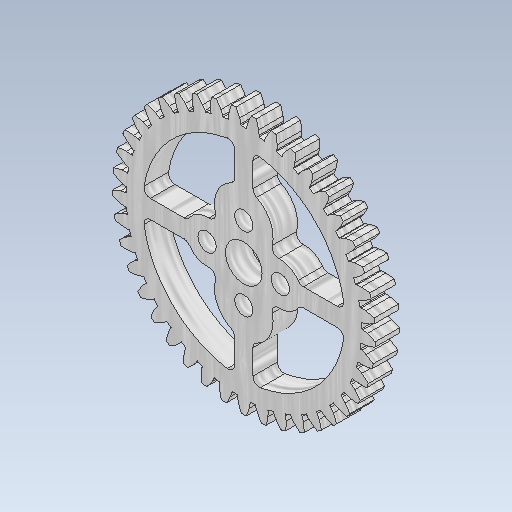
# Autodesk Inventor part: m1歯数41ギアd6t4
Saved by Autodesk Inventor 2020.2 (Build 242310000, 310)
## iProperties
Created: 2020-03-15
Part Number: m1歯数41ギアd6t4
Material: アルミニウム 7075
Document SubType Name: Modeling
Designer: aoyam
Density: 2.81 g/cm^3
Appearance: サテン - ブラシ仕上げ 重厚
Mass: 7.9651 g
Surface Area: 34.7064 cm^2
Volume: 2.83456 cm^3
Author: aoyam
Autodesk Inventor part; units mm, degrees
ref_plane "YZ Plane" through (0, 0, 0) normal (1, 0, 0) x (0, 1, 0)
ref_plane "XZ Plane" through (0, 0, 0) normal (0, 1, 0) x (-1, 0, 0)
ref_plane "XY Plane" through (0, 0, 0) normal (0, 0, 1) x (1, 0, 0)
sketch "スケッチ1" plane through (0, 0, 0) normal (0, 0, 1) x (1, 0, 0)
  arc A0 (3.2074, 20.8841) -> (3.1784, 20.6559) centre (4.8478, 20.5595) ccw
  arc A1 (3.4025, 21.5932) -> (3.2074, 20.8841) centre (7.7041, 20.0288) ccw
  arc A2 (3.993, 22.8602) -> (3.4025, 21.5932) centre (10.7748, 18.928) ccw
  arc A3 (2.2767, 20.6559) -> (2.2477, 20.8841) centre (0.6073, 20.5595) ccw
  arc A4 (2.2477, 20.8841) -> (2.0526, 21.5932) centre (-2.249, 20.0288) ccw
  arc A5 (2.0526, 21.5932) -> (1.4621, 22.8602) centre (-5.3197, 18.928) ccw
  arc A6 (3.1781, 20.6422) -> (2.277, 20.6422) centre (2.7276, 1.3974) ccw
  arc A7 (1.4621, 22.8602) -> (0.7019, 22.8018) centre (2.7276, 1.3974) ccw
  line L0 (3.1781, 20.6422) -> (3.1784, 20.6559)
  line L1 (2.277, 20.6422) -> (2.2767, 20.6559)
  arc A8 (0.2272, 20.729) -> (0.2334, 20.499) centre (1.8978, 20.6586) ccw
  arc A9 (0.2351, 20.4854) -> (-0.6554, 20.3478) centre (2.7276, 1.3974) ccw
  line L2 (0.2351, 20.4854) -> (0.2334, 20.499)
  line L3 (-0.6554, 20.3478) -> (-0.6578, 20.3613)
  arc A10 (-0.6578, 20.3613) -> (-0.7213, 20.5824) centre (-2.2929, 20.0113) ccw
  arc A11 (0.3117, 21.4596) -> (0.2272, 20.729) centre (4.8017, 20.5701) ccw
  arc A12 (-0.7213, 20.5824) -> (-1.0223, 21.2535) centre (-5.0348, 19.0507) ccw
  arc A13 (0.7019, 22.8018) -> (0.3117, 21.4596) centre (8.0044, 19.9509) ccw
  arc A14 (-1.0223, 21.2535) -> (-1.7994, 22.4155) centre (-7.9014, 17.4941) ccw
  arc A15 (-1.7994, 22.4155) -> (-2.5417, 22.2417) centre (2.7276, 1.3974) ccw
  arc A16 (-2.6944, 20.1207) -> (-2.6532, 19.8944) centre (-1.0326, 20.3062) ccw
  arc A17 (-2.6494, 19.8812) -> (-3.5085, 19.6093) centre (2.7276, 1.3974) ccw
  line L4 (-2.6494, 19.8812) -> (-2.6532, 19.8944)
  line L5 (-3.5085, 19.6093) -> (-3.513, 19.6223)
  arc A18 (-3.513, 19.6223) -> (-3.6095, 19.8311) centre (-5.0755, 19.0268) ccw
  arc A19 (-2.7225, 20.8557) -> (-2.6944, 20.1207) centre (1.8507, 20.662) ccw
  arc A20 (-3.6095, 19.8311) -> (-4.0094, 20.4484) centre (-7.6385, 17.6589) ccw
  arc A21 (-2.5417, 22.2417) -> (-2.7225, 20.8557) centre (5.1104, 20.539) ccw
  arc A22 (-4.0094, 20.4484) -> (-4.9547, 21.4781) centre (-10.234, 15.683) ccw
  arc A23 (-4.9547, 21.4781) -> (-5.6618, 21.1931) centre (2.7276, 1.3974) ccw
  arc A24 (-5.489, 19.0736) -> (-5.4137, 18.8562) centre (-3.875, 19.5106) ccw
  arc A25 (-5.4079, 18.8438) -> (-6.2155, 18.444) centre (2.7276, 1.3974) ccw
  line L6 (-5.4079, 18.8438) -> (-5.4137, 18.8562)
  line L7 (-6.2155, 18.444) -> (-6.2219, 18.4561)
  arc A26 (-6.2219, 18.4561) -> (-6.3491, 18.6477) centre (-7.6751, 17.6291) ccw
  arc A27 (-5.6289, 19.7957) -> (-5.489, 19.0736) centre (-1.0797, 20.3024) ccw
  arc A28 (-6.3491, 18.6477) -> (-6.8386, 19.1967) centre (-9.9994, 15.886) ccw
  arc A29 (-5.6618, 21.1931) -> (-5.6289, 19.7957) centre (2.1605, 20.6784) ccw
  arc A30 (-6.8386, 19.1967) -> (-7.93, 20.0701) centre (-12.2627, 13.537) ccw
  arc A31 (-7.93, 20.0701) -> (-8.5853, 19.6805) centre (2.7276, 1.3974) ccw
  arc A32 (-8.091, 17.6122) -> (-7.9834, 17.4089) centre (-6.5626, 18.2905) ccw
  arc A33 (-7.9758, 17.3975) -> (-8.7128, 16.879) centre (2.7276, 1.3974) ccw
  line L8 (-7.9758, 17.3975) -> (-7.9834, 17.4089)
  line L9 (-8.7128, 16.879) -> (-8.721, 16.8901)
  arc A34 (-8.721, 16.8901) -> (-8.876, 17.06) centre (-10.031, 15.8509) ccw
  arc A35 (-8.3394, 18.3045) -> (-8.091, 17.6122) centre (-3.9209, 19.4997) ccw
  arc A36 (-8.876, 17.06) -> (-9.4435, 17.5279) centre (-12.0619, 13.7734) ccw
  arc A37 (-8.5853, 19.6805) -> (-8.3394, 18.3045) centre (-0.7761, 20.3659) ccw
  arc A38 (-9.4435, 17.5279) -> (-10.6554, 18.2244) centre (-13.9401, 11.1065) ccw
  arc A39 (-10.6554, 18.2244) -> (-11.2436, 17.7393) centre (2.7276, 1.3974) ccw
  arc A40 (-10.4393, 15.7708) -> (-10.302, 15.5862) centre (-9.0324, 16.6744) ccw
  arc A41 (-10.2927, 15.5761) -> (-10.942, 14.9512) centre (2.7276, 1.3974) ccw
  line L10 (-10.2927, 15.5761) -> (-10.302, 15.5862)
  line L11 (-10.942, 14.9512) -> (-10.9517, 14.9609)
  arc A42 (-10.9517, 14.9609) -> (-11.1309, 15.1052) centre (-12.0877, 13.7339) ccw
  arc A43 (-10.7906, 16.417) -> (-10.4393, 15.7708) centre (-6.6063, 18.2726) ccw
  arc A44 (-11.1309, 15.1052) -> (-11.7632, 15.4809) centre (-13.7777, 11.3708) ccw
  arc A45 (-11.2436, 17.7393) -> (-10.7906, 16.417) centre (-3.6305, 19.6088) ccw
  arc A46 (-11.7632, 15.4809) -> (-13.0672, 15.9843) centre (-15.2269, 8.4484) ccw
  arc A47 (-13.0672, 15.9843) -> (-13.5744, 15.4151) centre (2.7276, 1.3974) ccw
  arc A48 (-12.4791, 13.5924) -> (-12.3152, 13.431) centre (-11.2266, 14.7002) ccw
  arc A49 (-12.3045, 13.4224) -> (-12.8508, 12.7058) centre (2.7276, 1.3974) ccw
  line L12 (-12.3045, 13.4224) -> (-12.3152, 13.431)
  line L13 (-12.8508, 12.7058) -> (-12.8619, 12.7138)
  arc A50 (-12.8619, 12.7138) -> (-13.061, 12.8291) centre (-13.7973, 11.3278) ccw
  arc A51 (-12.9249, 14.1774) -> (-12.4791, 13.5924) centre (-9.0729, 16.65) ccw
  arc A52 (-13.061, 12.8291) -> (-13.7432, 13.1039) centre (-15.1067, 8.7344) ccw
  arc A53 (-13.5744, 15.4151) -> (-12.9249, 14.1774) centre (-6.336, 18.4248) ccw
  arc A54 (-13.7432, 13.1039) -> (-15.1088, 13.4023) centre (-16.0928, 5.625) ccw
  arc A55 (-15.1088, 13.4023) -> (-15.5232, 12.7623) centre (2.7276, 1.3974) ccw
  arc A56 (-14.1624, 11.1282) -> (-13.9758, 10.9937) centre (-13.0937, 12.4142) ccw
  arc A57 (-13.9639, 10.9868) -> (-14.3944, 10.1952) centre (2.7276, 1.3974) ccw
  line L14 (-13.9639, 10.9868) -> (-13.9758, 10.9937)
  line L15 (-14.3944, 10.1952) -> (-14.4066, 10.2015)
  arc A58 (-14.4066, 10.2015) -> (-14.621, 10.285) centre (-15.1195, 8.6889) ccw
  arc A59 (-14.6923, 11.6383) -> (-14.1624, 11.1282) centre (-11.2629, 14.67) ccw
  arc A60 (-14.621, 10.285) -> (-15.3371, 10.4524) centre (-16.0177, 5.926) ccw
  arc A61 (-15.5232, 12.7623) -> (-14.6923, 11.6383) centre (-8.8289, 16.8417) ccw
  arc A62 (-15.3371, 10.4524) -> (-16.7323, 10.5389) centre (-16.5176, 2.7026) ccw
  arc A63 (-16.7323, 10.5389) -> (-17.0441, 9.8432) centre (2.7276, 1.3974) ccw
  arc A64 (-15.4499, 8.4359) -> (-15.2449, 8.3314) centre (-14.59, 9.87) ccw
  arc A65 (-15.2321, 8.3265) -> (-15.5367, 7.4784) centre (2.7276, 1.3974) ccw
  line L16 (-15.2321, 8.3265) -> (-15.2449, 8.3314)
  line L17 (-15.5367, 7.4784) -> (-15.5497, 7.4828)
  arc A66 (-15.5497, 7.4828) -> (-15.7743, 7.5326) centre (-16.0233, 5.8791) ccw
  arc A67 (-16.0514, 8.8592) -> (-15.4499, 8.4359) centre (-13.125, 12.3788) ccw
  arc A68 (-15.7743, 7.5326) -> (-16.5077, 7.5887) centre (-16.4893, 3.0115) ccw
  arc A69 (-17.0441, 9.8432) -> (-16.0514, 8.8592) centre (-11.0511, 14.8966) ccw
  arc A70 (-16.5077, 7.5887) -> (-17.8996, 7.4612) centre (-16.4912, -0.2505) ccw
  arc A71 (-17.8996, 7.4612) -> (-18.1017, 6.7261) centre (2.7276, 1.3974) ccw
  arc A72 (-16.3113, 5.5786) -> (-16.0928, 5.5067) centre (-15.6804, 7.1272) ccw
  arc A73 (-16.0794, 5.5038) -> (-16.2509, 4.6191) centre (2.7276, 1.3974) ccw
  line L18 (-16.0794, 5.5038) -> (-16.0928, 5.5067)
  line L19 (-16.2509, 4.6191) -> (-16.2644, 4.6214)
  arc A74 (-16.2644, 4.6214) -> (-16.494, 4.6364) centre (-16.4877, 2.9643) ccw
  arc A75 (-16.9703, 5.9051) -> (-16.3113, 5.5786) centre (-14.6155, 9.8302) ccw
  arc A76 (-16.494, 4.6364) -> (-17.2273, 4.5799) centre (-16.5105, 0.0591) ccw
  arc A77 (-18.1017, 6.7261) -> (-16.9703, 5.9051) centre (-12.9502, 12.6351) ccw
  arc A78 (-17.2273, 4.5799) -> (-18.5835, 4.2414) centre (-16.0145, -3.1649) ccw
  arc A79 (-18.5835, 4.2414) -> (-18.671, 3.4841) centre (2.7276, 1.3974) ccw
  arc A80 (-16.7264, 2.6234) -> (-16.4995, 2.5856) centre (-16.3393, 4.2501) ccw
  arc A81 (-16.4858, 2.5848) -> (-16.5203, 1.6843) centre (2.7276, 1.3974) ccw
  line L20 (-16.4858, 2.5848) -> (-16.4995, 2.5856)
  line L21 (-16.5203, 1.6843) -> (-16.534, 1.6845)
  arc A82 (-16.534, 1.6845) -> (-16.7632, 1.6643) centre (-16.5017, 0.0127) ccw
  arc A83 (-17.4276, 2.8454) -> (-16.7264, 2.6234) centre (-15.6995, 7.084) ccw
  arc A84 (-16.7632, 1.6643) -> (-17.4793, 1.4965) centre (-16.0807, -2.8619) ccw
  arc A85 (-18.671, 3.4841) -> (-17.4276, 2.8454) centre (-14.4819, 10.1102) ccw
  arc A86 (-17.4793, 1.4965) -> (-18.7679, 0.955) centre (-15.0984, -5.9724) ccw
  arc A87 (-18.7679, 0.955) -> (-18.7387, 0.1931) centre (2.7276, 1.3974) ccw
  arc A88 (-16.6856, -0.3606) -> (-16.4555, -0.3633) centre (-16.5513, 1.3061) ccw
  arc A89 (-16.4419, -0.362) -> (-16.3385, -1.2572) centre (2.7276, 1.3974) ccw
  line L22 (-16.4419, -0.362) -> (-16.4555, -0.3633)
  line L23 (-16.3385, -1.2572) -> (-16.3521, -1.2591)
  arc A90 (-16.3521, -1.2591) -> (-16.5755, -1.3141) centre (-16.065, -2.9064) ccw
  arc A91 (-17.4124, -0.2482) -> (-16.6856, -0.3606) centre (-16.3516, 4.2045) ccw
  arc A92 (-16.5755, -1.3141) -> (-17.2576, -1.5892) centre (-15.2101, -5.683) ccw
  arc A93 (-18.7387, 0.1931) -> (-17.4124, -0.2482) centre (-15.6102, 7.3811) ccw
  arc A94 (-17.2576, -1.5892) -> (-18.4484, -2.3211) centre (-13.7645, -8.6071) ccw
  arc A95 (-18.4484, -2.3211) -> (-18.3033, -3.0696) centre (2.7276, 1.3974) ccw
  arc A96 (-16.1897, -3.3034) -> (-15.9619, -3.2709) centre (-16.3114, -1.6357) ccw
  arc A97 (-15.9486, -3.2676) -> (-15.7099, -4.1365) centre (2.7276, 1.3974) ccw
  line L24 (-15.9486, -3.2676) -> (-15.9619, -3.2709)
  line L25 (-15.7099, -4.1365) -> (-15.723, -4.1405)
  arc A98 (-15.723, -4.1405) -> (-15.9353, -4.2289) centre (-15.1878, -5.7246) ccw
  arc A99 (-16.9252, -3.3033) -> (-16.1897, -3.3034) centre (-16.5565, 1.2592) ccw
  arc A100 (-15.9353, -4.2289) -> (-16.5675, -4.6049) centre (-13.9191, -8.3382) ccw
  arc A101 (-18.3033, -3.0696) -> (-16.9252, -3.3033) centre (-16.3087, 4.5117) ccw
  arc A102 (-16.5675, -4.6049) -> (-17.6326, -5.51) centre (-12.044, -11.0074) ccw
  arc A103 (-17.6326, -5.51) -> (-17.3749, -6.2275) centre (2.7276, 1.3974) ccw
  arc A104 (-15.2504, -6.136) -> (-15.0303, -6.0692) centre (-15.6253, -4.5065) ccw
  arc A105 (-15.0176, -6.0638) -> (-14.649, -6.8861) centre (2.7276, 1.3974) ccw
  line L26 (-15.0176, -6.0638) -> (-15.0303, -6.0692)
  line L27 (-14.649, -6.8861) -> (-14.6614, -6.892)
  arc A106 (-14.6614, -6.892) -> (-14.8578, -7.0118) centre (-13.8906, -8.3759) ccw
  arc A107 (-15.9773, -6.2482) -> (-15.2504, -6.136) centre (-16.3094, -1.6829) ccw
  arc A108 (-14.8578, -7.0118) -> (-15.4251, -7.4799) centre (-12.2378, -10.7652) ccw
  arc A109 (-17.3749, -6.2275) -> (-15.9773, -6.2482) centre (-16.561, 1.5693) ccw
  arc A110 (-15.4251, -7.4799) -> (-16.3396, -8.537) centre (-9.9773, -13.1169) ccw
  arc A111 (-16.3396, -8.537) -> (-15.9754, -9.2068) centre (2.7276, 1.3974) ccw
  arc A112 (-13.8897, -8.7921) -> (-13.6824, -8.6924) centre (-14.5089, -7.2388) ccw
  arc A113 (-13.6707, -8.6852) -> (-13.1809, -9.4416) centre (2.7276, 1.3974) ccw
  line L28 (-13.6707, -8.6852) -> (-13.6824, -8.6924)
  line L29 (-13.1809, -9.4416) -> (-13.1922, -9.4493)
  arc A114 (-13.1922, -9.4493) -> (-13.368, -9.5977) centre (-12.204, -10.7981) ccw
  arc A115 (-14.591, -9.0138) -> (-13.8897, -8.7921) centre (-15.616, -4.5528) ccw
  arc A116 (-13.368, -9.5977) -> (-13.8572, -10.1469) centre (-10.2058, -12.9071) ccw
  arc A117 (-15.9754, -9.2068) -> (-14.591, -9.0138) centre (-16.3612, -1.3771) ccw
  arc A118 (-13.8572, -10.1469) -> (-14.5996, -11.3312) centre (-7.6128, -14.8861) ccw
  arc A119 (-14.5996, -11.3312) -> (-14.1375, -11.9375) centre (2.7276, 1.3974) ccw
  arc A120 (-12.1395, -11.2093) -> (-11.9499, -11.0791) centre (-12.9886, -9.7688) ccw
  arc A121 (-11.9394, -11.0702) -> (-11.3399, -11.7429) centre (2.7276, 1.3974) ccw
  line L30 (-11.9394, -11.0702) -> (-11.9499, -11.0791)
  line L31 (-11.3399, -11.7429) -> (-11.3499, -11.7523)
  arc A122 (-11.3499, -11.7523) -> (-11.501, -11.9258) centre (-10.1674, -12.9345) ccw
  arc A123 (-12.7987, -11.5355) -> (-12.1395, -11.2093) centre (-14.4928, -7.2832) ccw
  arc A124 (-11.501, -11.9258) -> (-11.9006, -12.5432) centre (-7.8707, -14.7137) ccw
  arc A125 (-14.1375, -11.9375) -> (-12.7987, -11.5355) centre (-15.7139, -4.2584) ccw
  arc A126 (-11.9006, -12.5432) -> (-12.4536, -13.827) centre (-5.0059, -16.2738) ccw
  arc A127 (-12.4536, -13.827) -> (-11.9042, -14.3557) centre (2.7276, 1.3974) ccw
  arc A128 (-10.0409, -13.331) -> (-9.8733, -13.1734) centre (-11.0999, -12.037) ccw
  arc A129 (-9.8644, -13.163) -> (-9.1692, -13.7363) centre (2.7276, 1.3974) ccw
  line L32 (-9.8644, -13.163) -> (-9.8733, -13.1734)
  line L33 (-9.1692, -13.7363) -> (-9.1776, -13.7471)
  arc A130 (-9.1776, -13.7471) -> (-9.3004, -13.9416) centre (-7.8285, -14.7349) ccw
  arc A131 (-10.6426, -13.754) -> (-10.0409, -13.331) centre (-12.9659, -9.8101) ccw
  arc A132 (-9.3004, -13.9416) -> (-9.6012, -14.6128) centre (-5.2871, -16.1427) ccw
  arc A133 (-11.9042, -14.3557) -> (-10.6426, -13.754) centre (-14.6345, -7.0072) ccw
  arc A134 (-9.6012, -14.6128) -> (-9.9516, -15.966) centre (-2.2178, -17.2472) ccw
  arc A135 (-9.9516, -15.966) -> (-9.3281, -16.4046) centre (2.7276, 1.3974) ccw
  arc A136 (-7.643, -15.1074) -> (-7.5014, -14.9261) centre (-8.8871, -13.9903) ccw
  arc A137 (-7.4942, -14.9145) -> (-6.7196, -15.375) centre (2.7276, 1.3974) ccw
  line L34 (-7.4942, -14.9145) -> (-7.5014, -14.9261)
  line L35 (-6.7196, -15.375) -> (-6.7263, -15.3869)
  arc A138 (-6.7263, -15.3869) -> (-6.818, -15.5979) centre (-5.2422, -16.1572) ccw
  arc A139 (-8.173, -15.6173) -> (-7.643, -15.1074) centre (-11.0711, -12.0744) ccw
  arc A140 (-6.818, -15.5979) -> (-7.0127, -16.3072) centre (-2.5157, -17.1606) ccw
  arc A141 (-9.3281, -16.4046) -> (-8.173, -15.6173) centre (-13.148, -9.559) ccw
  arc A142 (-7.0127, -16.3072) -> (-7.1525, -17.698) centre (0.6862, -17.7836) ccw
  arc A143 (-7.1525, -17.698) -> (-6.4693, -18.0362) centre (2.7276, 1.3974) ccw
  arc A144 (-5.002, -16.4971) -> (-4.8898, -16.2963) centre (-6.4021, -15.5829) ccw
  arc A145 (-4.8844, -16.2837) -> (-4.0486, -16.6205) centre (2.7276, 1.3974) ccw
  line L36 (-4.8844, -16.2837) -> (-4.8898, -16.2963)
  line L37 (-4.0486, -16.6205) -> (-4.0534, -16.6333)
  arc A146 (-4.0534, -16.6333) -> (-4.1118, -16.8559) centre (-2.4691, -17.168) ccw
  arc A147 (-5.448, -17.0819) -> (-5.002, -16.4971) centre (-8.8529, -14.0228) ccw
  arc A148 (-4.1118, -16.8559) -> (-4.196, -17.5865) centre (0.3786, -17.7435) ccw
  arc A149 (-6.4693, -18.0362) -> (-5.448, -17.0819) centre (-11.2895, -11.854) ccw
  arc A150 (-4.196, -17.5865) -> (-4.1219, -18.9824) centre (3.6381, -17.8704) ccw
  arc A151 (-4.1219, -18.9824) -> (-3.395, -19.2124) centre (2.7276, 1.3974) ccw
  arc A152 (-2.1798, -17.4673) -> (-2.0996, -17.2517) centre (-3.703, -16.7775) ccw
  arc A153 (-2.0961, -17.2384) -> (-1.2187, -17.4437) centre (2.7276, 1.3974) ccw
  line L38 (-2.0961, -17.2384) -> (-2.0996, -17.2517)
  line L39 (-1.2187, -17.4437) -> (-1.2215, -17.4571)
  arc A154 (-1.2215, -17.4571) -> (-1.2453, -17.686) centre (0.4258, -17.7437) ccw
  arc A155 (-2.5313, -18.1133) -> (-2.1798, -17.4673) centre (-6.3633, -15.6099) ccw
  arc A156 (-1.2453, -17.686) -> (-1.217, -18.4209) centre (3.328, -17.8777) ccw
  arc A157 (-3.395, -19.2124) -> (-2.5313, -18.1133) centre (-9.1024, -13.8384) ccw
  arc A158 (-1.217, -18.4209) -> (-0.9306, -19.7891) centre (6.5687, -17.5056) ccw
  arc A159 (-0.9306, -19.7891) -> (-0.1772, -19.9054) centre (2.7276, 1.3974) ccw
  arc A160 (0.7574, -17.9953) -> (0.8038, -17.77) centre (-0.8533, -17.5461) ccw
  arc A161 (0.8051, -17.7563) -> (1.7036, -17.8253) centre (2.7276, 1.3974) ccw
  line L40 (0.8051, -17.7563) -> (0.8038, -17.77)
  line L41 (1.7036, -17.8253) -> (1.7029, -17.839)
  arc A162 (1.7029, -17.839) -> (1.7144, -18.0688) centre (3.3747, -17.8707) ccw
  arc A163 (0.5086, -18.6874) -> (0.7574, -17.9953) centre (-3.6606, -16.7983) ccw
  arc A164 (1.7144, -18.0688) -> (1.8545, -18.7908) centre (6.2633, -17.5602) ccw
  arc A165 (-0.1772, -19.9054) -> (0.5086, -18.6874) centre (-6.638, -15.4657) ccw
  arc A166 (1.8545, -18.7908) -> (2.3464, -20.0992) centre (9.4092, -16.6977) ccw
  arc A167 (2.3464, -20.0992) -> (3.1087, -20.0992) centre (2.7276, 1.3974) ccw
  arc A168 (3.7407, -18.0688) -> (3.7522, -17.839) centre (2.0804, -17.8707) ccw
  arc A169 (3.7515, -17.8253) -> (4.65, -17.7563) centre (2.7276, 1.3974) ccw
  line L42 (3.7515, -17.8253) -> (3.7522, -17.839)
  line L43 (4.65, -17.7563) -> (4.6513, -17.77)
  arc A170 (4.6513, -17.77) -> (4.6977, -17.9953) centre (6.3084, -17.5461) ccw
  arc A171 (3.6006, -18.7908) -> (3.7407, -18.0688) centre (-0.8082, -17.5602) ccw
  arc A172 (4.6977, -17.9953) -> (4.9465, -18.6874) centre (9.1157, -16.7983) ccw
  arc A173 (3.1087, -20.0992) -> (3.6006, -18.7908) centre (-3.9541, -16.6977) ccw
  arc A174 (4.9465, -18.6874) -> (5.6323, -19.9054) centre (12.0931, -15.4657) ccw
  arc A175 (5.6323, -19.9054) -> (6.3857, -19.7891) centre (2.7276, 1.3974) ccw
  arc A176 (6.7004, -17.686) -> (6.6766, -17.4571) centre (5.0293, -17.7437) ccw
  arc A177 (6.6738, -17.4437) -> (7.5512, -17.2384) centre (2.7276, 1.3974) ccw
  line L44 (6.6738, -17.4437) -> (6.6766, -17.4571)
  line L45 (7.5512, -17.2384) -> (7.5547, -17.2517)
  arc A178 (7.5547, -17.2517) -> (7.6349, -17.4673) centre (9.1581, -16.7775) ccw
  arc A179 (6.6721, -18.4209) -> (6.7004, -17.686) centre (2.1271, -17.8777) ccw
  arc A180 (7.6349, -17.4673) -> (7.9864, -18.1133) centre (11.8184, -15.6099) ccw
  arc A181 (6.3857, -19.7891) -> (6.6721, -18.4209) centre (-1.1136, -17.5056) ccw
  arc A182 (7.9864, -18.1133) -> (8.8501, -19.2124) centre (14.5575, -13.8384) ccw
  arc A183 (8.8501, -19.2124) -> (9.577, -18.9824) centre (2.7276, 1.3974) ccw
  arc A184 (9.5669, -16.8559) -> (9.5085, -16.6333) centre (7.9242, -17.168) ccw
  arc A185 (9.5037, -16.6205) -> (10.3395, -16.2837) centre (2.7276, 1.3974) ccw
  line L46 (9.5037, -16.6205) -> (9.5085, -16.6333)
  line L47 (10.3395, -16.2837) -> (10.3449, -16.2963)
  arc A186 (10.3449, -16.2963) -> (10.4571, -16.4971) centre (11.8572, -15.5829) ccw
  arc A187 (9.6511, -17.5865) -> (9.5669, -16.8559) centre (5.0765, -17.7435) ccw
  arc A188 (10.4571, -16.4971) -> (10.9031, -17.0819) centre (14.308, -14.0228) ccw
  arc A189 (9.577, -18.9824) -> (9.6511, -17.5865) centre (1.817, -17.8704) ccw
  arc A190 (10.9031, -17.0819) -> (11.9244, -18.0362) centre (16.7446, -11.854) ccw
  arc A191 (11.9244, -18.0362) -> (12.6076, -17.698) centre (2.7276, 1.3974) ccw
  arc A192 (12.2731, -15.5979) -> (12.1814, -15.3869) centre (10.6973, -16.1572) ccw
  arc A193 (12.1747, -15.375) -> (12.9493, -14.9145) centre (2.7276, 1.3974) ccw
  line L48 (12.1747, -15.375) -> (12.1814, -15.3869)
  line L49 (12.9493, -14.9145) -> (12.9565, -14.9261)
  arc A194 (12.9565, -14.9261) -> (13.0981, -15.1074) centre (14.3422, -13.9903) ccw
  arc A195 (12.4678, -16.3072) -> (12.2731, -15.5979) centre (7.9708, -17.1606) ccw
  arc A196 (13.0981, -15.1074) -> (13.6281, -15.6173) centre (16.5262, -12.0744) ccw
  arc A197 (12.6076, -17.698) -> (12.4678, -16.3072) centre (4.7689, -17.7836) ccw
  arc A198 (13.6281, -15.6173) -> (14.7832, -16.4046) centre (18.6031, -9.559) ccw
  arc A199 (14.7832, -16.4046) -> (15.4067, -15.966) centre (2.7276, 1.3974) ccw
  arc A200 (14.7555, -13.9416) -> (14.6327, -13.7471) centre (13.2836, -14.7349) ccw
  arc A201 (14.6243, -13.7363) -> (15.3195, -13.163) centre (2.7276, 1.3974) ccw
  line L50 (14.6243, -13.7363) -> (14.6327, -13.7471)
  line L51 (15.3195, -13.163) -> (15.3284, -13.1734)
  arc A202 (15.3284, -13.1734) -> (15.496, -13.331) centre (16.555, -12.037) ccw
  arc A203 (15.0563, -14.6128) -> (14.7555, -13.9416) centre (10.7422, -16.1427) ccw
  arc A204 (15.496, -13.331) -> (16.0977, -13.754) centre (18.421, -9.8101) ccw
  arc A205 (15.4067, -15.966) -> (15.0563, -14.6128) centre (7.6729, -17.2472) ccw
  arc A206 (16.0977, -13.754) -> (17.3593, -14.3557) centre (20.0896, -7.0072) ccw
  arc A207 (17.3593, -14.3557) -> (17.9087, -13.827) centre (2.7276, 1.3974) ccw
  arc A208 (16.9561, -11.9258) -> (16.805, -11.7523) centre (15.6225, -12.9345) ccw
  arc A209 (16.795, -11.7429) -> (17.3945, -11.0702) centre (2.7276, 1.3974) ccw
  line L52 (16.795, -11.7429) -> (16.805, -11.7523)
  line L53 (17.3945, -11.0702) -> (17.405, -11.0791)
  arc A210 (17.405, -11.0791) -> (17.5946, -11.2093) centre (18.4437, -9.7688) ccw
  arc A211 (17.3557, -12.5432) -> (16.9561, -11.9258) centre (13.3258, -14.7137) ccw
  arc A212 (17.5946, -11.2093) -> (18.2538, -11.5355) centre (19.9479, -7.2832) ccw
  arc A213 (17.9087, -13.827) -> (17.3557, -12.5432) centre (10.461, -16.2738) ccw
  arc A214 (18.2538, -11.5355) -> (19.5926, -11.9375) centre (21.169, -4.2584) ccw
  arc A215 (19.5926, -11.9375) -> (20.0547, -11.3312) centre (2.7276, 1.3974) ccw
  arc A216 (18.8231, -9.5977) -> (18.6473, -9.4493) centre (17.6591, -10.7981) ccw
  arc A217 (18.636, -9.4416) -> (19.1258, -8.6852) centre (2.7276, 1.3974) ccw
  line L54 (18.636, -9.4416) -> (18.6473, -9.4493)
  line L55 (19.1258, -8.6852) -> (19.1375, -8.6924)
  arc A218 (19.1375, -8.6924) -> (19.3448, -8.7921) centre (19.964, -7.2388) ccw
  arc A219 (19.3123, -10.1469) -> (18.8231, -9.5977) centre (15.6609, -12.9071) ccw
  arc A220 (19.3448, -8.7921) -> (20.0461, -9.0138) centre (21.0711, -4.5528) ccw
  arc A221 (20.0547, -11.3312) -> (19.3123, -10.1469) centre (13.0679, -14.8861) ccw
  arc A222 (20.0461, -9.0138) -> (21.4305, -9.2068) centre (21.8163, -1.3771) ccw
  arc A223 (21.4305, -9.2068) -> (21.7947, -8.537) centre (2.7276, 1.3974) ccw
  arc A224 (20.3129, -7.0118) -> (20.1165, -6.892) centre (19.3457, -8.3759) ccw
  arc A225 (20.1041, -6.8861) -> (20.4727, -6.0638) centre (2.7276, 1.3974) ccw
  line L56 (20.1041, -6.8861) -> (20.1165, -6.892)
  line L57 (20.4727, -6.0638) -> (20.4854, -6.0692)
  arc A226 (20.4854, -6.0692) -> (20.7055, -6.136) centre (21.0804, -4.5065) ccw
  arc A227 (20.8802, -7.4799) -> (20.3129, -7.0118) centre (17.6929, -10.7652) ccw
  arc A228 (20.7055, -6.136) -> (21.4324, -6.2482) centre (21.7645, -1.6829) ccw
  arc A229 (21.7947, -8.537) -> (20.8802, -7.4799) centre (15.4324, -13.1169) ccw
  arc A230 (21.4324, -6.2482) -> (22.83, -6.2275) centre (22.0161, 1.5693) ccw
  arc A231 (22.83, -6.2275) -> (23.0877, -5.51) centre (2.7276, 1.3974) ccw
  arc A232 (21.3904, -4.2289) -> (21.1781, -4.1405) centre (20.6429, -5.7246) ccw
  arc A233 (21.165, -4.1365) -> (21.4037, -3.2676) centre (2.7276, 1.3974) ccw
  line L58 (21.165, -4.1365) -> (21.1781, -4.1405)
  line L59 (21.4037, -3.2676) -> (21.417, -3.2709)
  arc A234 (21.417, -3.2709) -> (21.6448, -3.3034) centre (21.7665, -1.6357) ccw
  arc A235 (22.0226, -4.6049) -> (21.3904, -4.2289) centre (19.3742, -8.3382) ccw
  arc A236 (21.6448, -3.3034) -> (22.3803, -3.3033) centre (22.0116, 1.2592) ccw
  arc A237 (23.0877, -5.51) -> (22.0226, -4.6049) centre (17.4991, -11.0074) ccw
  arc A238 (22.3803, -3.3033) -> (23.7584, -3.0696) centre (21.7638, 4.5117) ccw
  arc A239 (23.7584, -3.0696) -> (23.9035, -2.3211) centre (2.7276, 1.3974) ccw
  arc A240 (22.0306, -1.3141) -> (21.8072, -1.2591) centre (21.5201, -2.9064) ccw
  arc A241 (21.7936, -1.2572) -> (21.897, -0.362) centre (2.7276, 1.3974) ccw
  line L60 (21.7936, -1.2572) -> (21.8072, -1.2591)
  line L61 (21.897, -0.362) -> (21.9106, -0.3633)
  arc A242 (21.9106, -0.3633) -> (22.1407, -0.3606) centre (22.0064, 1.3061) ccw
  arc A243 (22.7127, -1.5892) -> (22.0306, -1.3141) centre (20.6652, -5.683) ccw
  arc A244 (22.1407, -0.3606) -> (22.8675, -0.2482) centre (21.8067, 4.2045) ccw
  arc A245 (23.9035, -2.3211) -> (22.7127, -1.5892) centre (19.2196, -8.6071) ccw
  arc A246 (22.8675, -0.2482) -> (24.1938, 0.1931) centre (21.0653, 7.3811) ccw
  arc A247 (24.1938, 0.1931) -> (24.223, 0.955) centre (2.7276, 1.3974) ccw
  arc A248 (22.2183, 1.6643) -> (21.9891, 1.6845) centre (21.9568, 0.0127) ccw
  arc A249 (21.9754, 1.6843) -> (21.9409, 2.5848) centre (2.7276, 1.3974) ccw
  line L62 (21.9754, 1.6843) -> (21.9891, 1.6845)
  line L63 (21.9409, 2.5848) -> (21.9546, 2.5856)
  arc A250 (21.9546, 2.5856) -> (22.1815, 2.6234) centre (21.7944, 4.2501) ccw
  arc A251 (22.9344, 1.4965) -> (22.2183, 1.6643) centre (21.5358, -2.8619) ccw
  arc A252 (22.1815, 2.6234) -> (22.8827, 2.8454) centre (21.1546, 7.084) ccw
  arc A253 (24.223, 0.955) -> (22.9344, 1.4965) centre (20.5535, -5.9724) ccw
  arc A254 (22.8827, 2.8454) -> (24.1261, 3.4841) centre (19.937, 10.1102) ccw
  arc A255 (24.1261, 3.4841) -> (24.0386, 4.2414) centre (2.7276, 1.3974) ccw
  arc A256 (21.9491, 4.6364) -> (21.7195, 4.6214) centre (21.9428, 2.9643) ccw
  arc A257 (21.706, 4.6191) -> (21.5345, 5.5038) centre (2.7276, 1.3974) ccw
  line L64 (21.706, 4.6191) -> (21.7195, 4.6214)
  line L65 (21.5345, 5.5038) -> (21.5479, 5.5067)
  arc A258 (21.5479, 5.5067) -> (21.7664, 5.5786) centre (21.1355, 7.1272) ccw
  arc A259 (22.6824, 4.5799) -> (21.9491, 4.6364) centre (21.9656, 0.0591) ccw
  arc A260 (21.7664, 5.5786) -> (22.4254, 5.9051) centre (20.0706, 9.8302) ccw
  arc A261 (24.0386, 4.2414) -> (22.6824, 4.5799) centre (21.4696, -3.1649) ccw
  arc A262 (22.4254, 5.9051) -> (23.5568, 6.7261) centre (18.4053, 12.6351) ccw
  arc A263 (23.5568, 6.7261) -> (23.3547, 7.4612) centre (2.7276, 1.3974) ccw
  arc A264 (21.2294, 7.5326) -> (21.0048, 7.4828) centre (21.4784, 5.8791) ccw
  arc A265 (20.9918, 7.4784) -> (20.6872, 8.3265) centre (2.7276, 1.3974) ccw
  line L66 (20.9918, 7.4784) -> (21.0048, 7.4828)
  line L67 (20.6872, 8.3265) -> (20.7, 8.3314)
  arc A266 (20.7, 8.3314) -> (20.905, 8.4359) centre (20.0451, 9.87) ccw
  arc A267 (21.9628, 7.5887) -> (21.2294, 7.5326) centre (21.9444, 3.0115) ccw
  arc A268 (20.905, 8.4359) -> (21.5065, 8.8592) centre (18.5801, 12.3788) ccw
  arc A269 (23.3547, 7.4612) -> (21.9628, 7.5887) centre (21.9463, -0.2505) ccw
  arc A270 (21.5065, 8.8592) -> (22.4992, 9.8432) centre (16.5062, 14.8966) ccw
  arc A271 (22.4992, 9.8432) -> (22.1874, 10.5389) centre (2.7276, 1.3974) ccw
  arc A272 (20.0761, 10.285) -> (19.8617, 10.2015) centre (20.5746, 8.6889) ccw
  arc A273 (19.8495, 10.1952) -> (19.419, 10.9868) centre (2.7276, 1.3974) ccw
  line L68 (19.8495, 10.1952) -> (19.8617, 10.2015)
  line L69 (19.419, 10.9868) -> (19.4309, 10.9937)
  arc A274 (19.4309, 10.9937) -> (19.6175, 11.1282) centre (18.5488, 12.4142) ccw
  arc A275 (20.7922, 10.4524) -> (20.0761, 10.285) centre (21.4728, 5.926) ccw
  arc A276 (19.6175, 11.1282) -> (20.1474, 11.6383) centre (16.718, 14.67) ccw
  arc A277 (22.1874, 10.5389) -> (20.7922, 10.4524) centre (21.9727, 2.7026) ccw
  arc A278 (20.1474, 11.6383) -> (20.9783, 12.7623) centre (14.284, 16.8417) ccw
  arc A279 (20.9783, 12.7623) -> (20.5639, 13.4023) centre (2.7276, 1.3974) ccw
  arc A280 (18.5161, 12.8291) -> (18.317, 12.7138) centre (19.2524, 11.3278) ccw
  arc A281 (18.3059, 12.7058) -> (17.7596, 13.4224) centre (2.7276, 1.3974) ccw
  line L70 (18.3059, 12.7058) -> (18.317, 12.7138)
  line L71 (17.7596, 13.4224) -> (17.7703, 13.431)
  arc A282 (17.7703, 13.431) -> (17.9342, 13.5924) centre (16.6817, 14.7002) ccw
  arc A283 (19.1983, 13.1039) -> (18.5161, 12.8291) centre (20.5618, 8.7344) ccw
  arc A284 (17.9342, 13.5924) -> (18.38, 14.1774) centre (14.528, 16.65) ccw
  arc A285 (20.5639, 13.4023) -> (19.1983, 13.1039) centre (21.5479, 5.625) ccw
  arc A286 (18.38, 14.1774) -> (19.0295, 15.4151) centre (11.7911, 18.4248) ccw
  arc A287 (19.0295, 15.4151) -> (18.5223, 15.9843) centre (2.7276, 1.3974) ccw
  arc A288 (16.586, 15.1052) -> (16.4068, 14.9609) centre (17.5428, 13.7339) ccw
  arc A289 (16.3971, 14.9512) -> (15.7478, 15.5761) centre (2.7276, 1.3974) ccw
  line L72 (16.3971, 14.9512) -> (16.4068, 14.9609)
  line L73 (15.7478, 15.5761) -> (15.7571, 15.5862)
  arc A290 (15.7571, 15.5862) -> (15.8944, 15.7708) centre (14.4875, 16.6744) ccw
  arc A291 (17.2183, 15.4809) -> (16.586, 15.1052) centre (19.2328, 11.3708) ccw
  arc A292 (15.8944, 15.7708) -> (16.2457, 16.417) centre (12.0614, 18.2726) ccw
  arc A293 (18.5223, 15.9843) -> (17.2183, 15.4809) centre (20.682, 8.4484) ccw
  arc A294 (16.2457, 16.417) -> (16.6987, 17.7393) centre (9.0856, 19.6088) ccw
  arc A295 (16.6987, 17.7393) -> (16.1105, 18.2244) centre (2.7276, 1.3974) ccw
  arc A296 (14.3311, 17.06) -> (14.1761, 16.8901) centre (15.4861, 15.8509) ccw
  arc A297 (14.1679, 16.879) -> (13.4309, 17.3975) centre (2.7276, 1.3974) ccw
  line L74 (14.1679, 16.879) -> (14.1761, 16.8901)
  line L75 (13.4309, 17.3975) -> (13.4385, 17.4089)
  arc A298 (13.4385, 17.4089) -> (13.5461, 17.6122) centre (12.0177, 18.2905) ccw
  arc A299 (14.8986, 17.5279) -> (14.3311, 17.06) centre (17.517, 13.7734) ccw
  arc A300 (13.5461, 17.6122) -> (13.7945, 18.3045) centre (9.376, 19.4997) ccw
  arc A301 (16.1105, 18.2244) -> (14.8986, 17.5279) centre (19.3952, 11.1065) ccw
  arc A302 (13.7945, 18.3045) -> (14.0404, 19.6805) centre (6.2312, 20.3659) ccw
  arc A303 (14.0404, 19.6805) -> (13.3851, 20.0701) centre (2.7276, 1.3974) ccw
  arc A304 (11.8042, 18.6477) -> (11.677, 18.4561) centre (13.1302, 17.6291) ccw
  arc A305 (11.6706, 18.444) -> (10.863, 18.8438) centre (2.7276, 1.3974) ccw
  line L76 (11.6706, 18.444) -> (11.677, 18.4561)
  line L77 (10.863, 18.8438) -> (10.8688, 18.8562)
  arc A306 (10.8688, 18.8562) -> (10.9441, 19.0736) centre (9.3301, 19.5106) ccw
  arc A307 (12.2937, 19.1967) -> (11.8042, 18.6477) centre (15.4545, 15.886) ccw
  arc A308 (10.9441, 19.0736) -> (11.084, 19.7957) centre (6.5348, 20.3024) ccw
  arc A309 (13.3851, 20.0701) -> (12.2937, 19.1967) centre (17.7178, 13.537) ccw
  arc A310 (11.084, 19.7957) -> (11.1169, 21.1931) centre (3.2946, 20.6784) ccw
  arc A311 (11.1169, 21.1931) -> (10.4098, 21.4781) centre (2.7276, 1.3974) ccw
  arc A312 (9.0646, 19.8311) -> (8.9681, 19.6223) centre (10.5306, 19.0268) ccw
  arc A313 (8.9636, 19.6093) -> (8.1045, 19.8812) centre (2.7276, 1.3974) ccw
  line L78 (8.9636, 19.6093) -> (8.9681, 19.6223)
  line L79 (8.1045, 19.8812) -> (8.1083, 19.8944)
  arc A314 (8.1083, 19.8944) -> (8.1495, 20.1207) centre (6.4878, 20.3062) ccw
  arc A315 (9.4645, 20.4484) -> (9.0646, 19.8311) centre (13.0936, 17.6589) ccw
  arc A316 (8.1495, 20.1207) -> (8.1776, 20.8557) centre (3.6044, 20.662) ccw
  arc A317 (10.4098, 21.4781) -> (9.4645, 20.4484) centre (15.6891, 15.683) ccw
  arc A318 (8.1776, 20.8557) -> (7.9968, 22.2417) centre (0.3447, 20.539) ccw
  arc A319 (7.9968, 22.2417) -> (7.2545, 22.4155) centre (2.7276, 1.3974) ccw
  arc A320 (6.1764, 20.5824) -> (6.1129, 20.3613) centre (7.748, 20.0113) ccw
  arc A321 (6.1105, 20.3478) -> (5.22, 20.4854) centre (2.7276, 1.3974) ccw
  line L80 (6.1105, 20.3478) -> (6.1129, 20.3613)
  line L81 (5.22, 20.4854) -> (5.2217, 20.499)
  arc A322 (5.2217, 20.499) -> (5.2279, 20.729) centre (3.5573, 20.6586) ccw
  arc A323 (6.4774, 21.2535) -> (6.1764, 20.5824) centre (10.4899, 19.0507) ccw
  arc A324 (5.2279, 20.729) -> (5.1434, 21.4596) centre (0.6534, 20.5701) ccw
  arc A325 (7.2545, 22.4155) -> (6.4774, 21.2535) centre (13.3565, 17.4941) ccw
  arc A326 (5.1434, 21.4596) -> (4.7532, 22.8018) centre (-2.5493, 19.9509) ccw
  arc A327 (4.7532, 22.8018) -> (3.993, 22.8602) centre (2.7276, 1.3974) ccw
  circle A328 centre (2.7276, 1.3974) radius 2.99
  line L82 (2.7276, 1.3974) -> (2.7276, 7.3974)
  circle A329 centre (2.7276, 7.3974) radius 1.5
  line L83 (2.7276, 1.3974) -> (8.7276, 1.3974)
  circle A330 centre (8.7276, 1.3974) radius 1.495
  circle A331 centre (2.7276, -4.6026) radius 1.5
  circle A332 centre (-3.2724, 1.3974) radius 1.495
  circle A333 centre (2.7276, 7.3974) radius 2.8
  circle A334 centre (2.7276, -4.6026) radius 2.8
  circle A335 centre (2.7276, 1.3974) radius 19.25
  circle A336 centre (2.7276, 7.3974) radius 4.8
  circle A337 centre (2.7276, -4.6026) radius 4.8
  circle A338 centre (-3.2724, 1.3974) radius 3.495
  circle A339 centre (8.7276, 1.3974) radius 3.495
  circle A340 centre (2.7276, 1.3974) radius 16.55
  line L84 (2.7276, 7.3974) -> (2.7276, 17.9474) construction
  line L85 (4.2276, 7.3974) -> (4.2276, 17.9474)
  line L86 (1.2276, 17.9474) -> (1.2276, 7.3974)
  arc A341 (1.2276, 7.3974) -> (4.2276, 7.3974) centre (2.7276, 7.3974) ccw
  arc A342 (4.2276, 17.9474) -> (1.2276, 17.9474) centre (2.7276, 17.9474) ccw
  line L87 (-3.2724, 1.3974) -> (-13.8224, 1.3974) construction
  line L88 (-3.2724, 2.8974) -> (-13.8224, 2.8974)
  line L89 (-13.8224, -0.1026) -> (-3.2724, -0.1026)
  arc A343 (-3.2724, -0.1026) -> (-3.2724, 2.8974) centre (-3.2724, 1.3974) ccw
  arc A344 (-13.8224, 2.8974) -> (-13.8224, -0.1026) centre (-13.8224, 1.3974) ccw
  line L90 (2.7276, -4.6026) -> (2.7276, -15.1526) construction
  line L91 (1.2276, -4.6026) -> (1.2276, -15.1526)
  line L92 (4.2276, -15.1526) -> (4.2276, -4.6026)
  arc A345 (4.2276, -4.6026) -> (1.2276, -4.6026) centre (2.7276, -4.6026) ccw
  arc A346 (1.2276, -15.1526) -> (4.2276, -15.1526) centre (2.7276, -15.1526) ccw
  line L93 (8.7276, 1.3974) -> (19.2776, 1.3974) construction
  line L94 (8.7276, -0.1026) -> (19.2776, -0.1026)
  line L95 (19.2776, 2.8974) -> (8.7276, 2.8974)
  arc A347 (8.7276, 2.8974) -> (8.7276, -0.1026) centre (8.7276, 1.3974) ccw
  arc A348 (19.2776, -0.1026) -> (19.2776, 2.8974) centre (19.2776, 1.3974) ccw
  circle A349 centre (-2.9354, 5.9299) radius 1.05
  circle A350 centre (8.3905, 5.9299) radius 1.05
  circle A351 centre (8.3905, -3.1351) radius 1.05
  circle A352 centre (-2.9354, -3.1351) radius 1.05
  point P0 (0, 0)
  point P1 (14.6243, -13.7363)
  point P2 (15.3195, -13.163)
  point P3 (15.496, -13.331)
  point P4 (16.0977, -13.754)
  point P5 (17.3593, -14.3557)
  point P6 (17.9087, -13.827)
  point P7 (17.3557, -12.5432)
  point P8 (16.9561, -11.9258)
  point P9 (17.405, -11.0791)
  point P10 (17.5946, -11.2093)
  point P11 (18.2538, -11.5355)
  point P12 (19.5926, -11.9375)
  point P13 (20.0547, -11.3312)
  point P14 (19.3123, -10.1469)
  point P15 (18.8231, -9.5977)
  point P16 (18.636, -9.4416)
  point P17 (19.1258, -8.6852)
  point P18 (19.3448, -8.7921)
  point P19 (20.0461, -9.0138)
  point P20 (21.4305, -9.2068)
  point P21 (21.7947, -8.537)
  point P22 (20.8802, -7.4799)
  point P23 (20.3129, -7.0118)
  point P24 (20.1165, -6.892)
  point P25 (20.1041, -6.8861)
  point P26 (20.4727, -6.0638)
  point P27 (20.7055, -6.136)
  point P28 (21.4324, -6.2482)
  point P29 (22.83, -6.2275)
  point P30 (23.0877, -5.51)
  point P31 (22.0226, -4.6049)
  point P32 (21.3904, -4.2289)
  point P33 (21.1781, -4.1405)
  point P34 (21.165, -4.1365)
  point P35 (21.4037, -3.2676)
  point P36 (21.6448, -3.3034)
  point P37 (22.3803, -3.3033)
  point P38 (23.7584, -3.0696)
  point P39 (23.9035, -2.3211)
  point P40 (22.7127, -1.5892)
  point P41 (22.0306, -1.3141)
  point P42 (21.8072, -1.2591)
  point P43 (21.7936, -1.2572)
  point P44 (21.897, -0.362)
  point P45 (22.1407, -0.3606)
  point P46 (22.8675, -0.2482)
  point P47 (24.1938, 0.1931)
  point P48 (24.223, 0.955)
  point P49 (22.9344, 1.4965)
  point P50 (22.2183, 1.6643)
  point P51 (21.9891, 1.6845)
  point P52 (21.9754, 1.6843)
  point P53 (21.9409, 2.5848)
  point P54 (22.1815, 2.6234)
  point P55 (22.8827, 2.8454)
  point P56 (24.1261, 3.4841)
  point P57 (24.0386, 4.2414)
  point P58 (22.6824, 4.5799)
  point P59 (21.9491, 4.6364)
  point P60 (21.7195, 4.6214)
  point P61 (21.706, 4.6191)
  point P62 (21.5345, 5.5038)
  point P63 (21.7664, 5.5786)
  point P64 (22.4254, 5.9051)
  point P65 (23.5568, 6.7261)
  point P66 (23.3547, 7.4612)
  point P67 (21.9628, 7.5887)
  point P68 (21.2294, 7.5326)
  point P69 (21.0048, 7.4828)
  point P70 (20.9918, 7.4784)
  point P71 (20.6872, 8.3265)
  point P72 (20.905, 8.4359)
  point P73 (22.4992, 9.8432)
  point P74 (22.1874, 10.5389)
  point P75 (20.7922, 10.4524)
  point P76 (20.0761, 10.285)
  point P77 (19.8617, 10.2015)
  point P78 (19.8495, 10.1952)
  point P79 (19.419, 10.9868)
  point P80 (19.6175, 11.1282)
  point P81 (20.1474, 11.6383)
  point P82 (20.9783, 12.7623)
  point P83 (20.5639, 13.4023)
  point P84 (19.1983, 13.1039)
  point P85 (18.5161, 12.8291)
  point P86 (18.317, 12.7138)
  point P87 (18.3059, 12.7058)
  point P88 (17.7596, 13.4224)
  point P89 (17.9342, 13.5924)
  point P90 (18.38, 14.1774)
  point P91 (19.0295, 15.4151)
  point P92 (18.5223, 15.9843)
  point P93 (17.2183, 15.4809)
  point P94 (16.586, 15.1052)
  point P95 (16.4068, 14.9609)
  point P96 (16.3971, 14.9512)
  point P97 (15.7478, 15.5761)
  point P98 (15.8944, 15.7708)
  point P99 (16.2457, 16.417)
  point P100 (16.6987, 17.7393)
  point P101 (16.1105, 18.2244)
  point P102 (14.8986, 17.5279)
  point P103 (14.3311, 17.06)
  point P104 (14.1679, 16.879)
  point P105 (13.4309, 17.3975)
  point P106 (13.5461, 17.6122)
  point P107 (13.7945, 18.3045)
  point P108 (14.0404, 19.6805)
  point P109 (13.3851, 20.0701)
  point P110 (12.2937, 19.1967)
  point P111 (11.8042, 18.6477)
  point P112 (11.677, 18.4561)
  point P113 (11.6706, 18.444)
  point P114 (10.863, 18.8438)
  point P115 (10.9441, 19.0736)
  point P116 (11.084, 19.7957)
  point P117 (11.1169, 21.1931)
  point P118 (9.4645, 20.4484)
  point P119 (9.0646, 19.8311)
  point P120 (8.1495, 20.1207)
  point P121 (8.1776, 20.8557)
  point P122 (7.9968, 22.2417)
  point P123 (7.2545, 22.4155)
  point P124 (6.4774, 21.2535)
  point P125 (6.1764, 20.5824)
  point P126 (6.1105, 20.3478)
  point P127 (5.22, 20.4854)
  point P128 (5.2279, 20.729)
  point P129 (5.1434, 21.4596)
  point P130 (4.7532, 22.8018)
  point P131 (3.993, 22.8602)
  point P132 (3.4025, 21.5932)
  point P133 (3.2074, 20.8841)
  point P134 (3.1784, 20.6559)
  point P135 (3.1781, 20.6422)
  point P136 (2.277, 20.6422)
  point P137 (2.2767, 20.6559)
  point P138 (2.2477, 20.8841)
  point P139 (2.0526, 21.5932)
  point P140 (1.4621, 22.8602)
  point P141 (0.7019, 22.8018)
  point P142 (0.3117, 21.4596)
  point P143 (0.2272, 20.729)
  point P144 (0.2334, 20.499)
  point P145 (0.2351, 20.4854)
  point P146 (-0.6578, 20.3613)
  point P147 (-0.7213, 20.5824)
  point P148 (-1.0223, 21.2535)
  point P149 (-1.7994, 22.4155)
  point P150 (-2.5417, 22.2417)
  point P151 (-2.7225, 20.8557)
  point P152 (-2.6944, 20.1207)
  point P153 (-3.513, 19.6223)
  point P154 (-3.6095, 19.8311)
  point P155 (-4.0094, 20.4484)
  point P156 (-4.9547, 21.4781)
  point P157 (-5.6618, 21.1931)
  point P158 (-5.6289, 19.7957)
  point P159 (-5.489, 19.0736)
  point P160 (-6.3491, 18.6477)
  point P161 (-6.8386, 19.1967)
  point P162 (-7.93, 20.0701)
  point P163 (-8.3394, 18.3045)
  point P164 (-8.091, 17.6122)
  point P165 (-8.7128, 16.879)
  point P166 (-8.876, 17.06)
  point P167 (-9.4435, 17.5279)
  point P168 (-10.6554, 18.2244)
  point P169 (-11.2436, 17.7393)
  point P170 (-10.4393, 15.7708)
  point P171 (-10.302, 15.5862)
  point P172 (-10.2927, 15.5761)
  point P173 (-10.942, 14.9512)
  point P174 (-11.1309, 15.1052)
  point P175 (-11.7632, 15.4809)
  point P176 (-13.0672, 15.9843)
  point P177 (-12.9249, 14.1774)
  point P178 (-12.4791, 13.5924)
  point P179 (-12.3152, 13.431)
  point P180 (-12.3045, 13.4224)
  point P181 (-12.8508, 12.7058)
  point P182 (-12.8619, 12.7138)
  point P183 (-13.061, 12.8291)
  point P184 (-15.1088, 13.4023)
  point P185 (-14.1624, 11.1282)
  point P186 (-13.9758, 10.9937)
  point P187 (-13.9639, 10.9868)
  point P188 (-14.4066, 10.2015)
  point P189 (-14.621, 10.285)
  point P190 (-16.7323, 10.5389)
  point P191 (-17.0441, 9.8432)
  point P192 (-15.4499, 8.4359)
  point P193 (-15.2449, 8.3314)
  point P194 (-15.2321, 8.3265)
  point P195 (-15.7743, 7.5326)
  point P196 (-16.5077, 7.5887)
  point P197 (-17.8996, 7.4612)
  point P198 (-18.1017, 6.7261)
  point P199 (-16.9703, 5.9051)
  dimension "d2" = 360
  dimension "d4" = 5.98
  dimension "d7" = 6
  dimension "d8" = 3
  dimension "d9" = 6
  dimension "d10" = 2.99
  dimension "d13" = 360
  dimension "d17" = 360
  dimension "d19" = 5.6
  dimension "d20" = 5.6
  dimension "d23" = 38.5
  dimension "d24" = 2
  dimension "d25" = 2
  dimension "d26" = 2
  dimension "d27" = 2
  dimension "d28" = 2.7
  dimension "d29" = 3
  dimension "d30" = 3
  dimension "d31" = 3
  dimension "d32" = 3
  dimension "d34" = 2.1
  dimension "d35" = 2.1
  dimension "d36" = 2.1
  dimension "d37" = 2.1
  constraints: 676 point on circle, 353 centre point, 200 end point, 24 tangent, 9 coincident, 4 midpoint, 4 parallel, 2 point on line, 1 perpendicular, 1 vertical, 1568 other
  measures "d4" diameter of A328
  measures "d7" distance of L82.start L82.end
  measures "d8" diameter of A329
  measures "d9" distance of L82.start L83.end
  measures "d10" diameter of A330
  measures "d19" diameter of A333
  measures "d20" diameter of A334
  measures "d23" diameter of A335
  measures "d24" radial gap between concentric circles of A333 A336
  measures "d25" radial gap between concentric circles of A334 A337
  measures "d26" radial gap between concentric circles of A332 A338
  measures "d27" radial gap between concentric circles of A330 A339
  measures "d28" radial gap between concentric circles of A340 A335
  measures "d29" diameter of A342
  measures "d30" diameter of A344
  measures "d31" diameter of A346
  measures "d32" diameter of A348
  measures "d34" diameter of A349
  measures "d35" diameter of A350
  measures "d36" diameter of A351
  measures "d37" diameter of A352
extrude "押し出し1" add sketch "スケッチ1" along normal blind 4 contours A1 A2 A327 A326 A324 A322 L81 A335 L0 A0 | A335 A321 A313 A305 A297 A289 A281 A273 A265 A257 A249 A241 A233 A225 A217 A209 A201 A193 A185 A177 A169 A161 A153 A145 A137 A129 A121 A113 A105 A97 A89 A81 A73 A65 A57 A49 A41 A33 A25 A17 A9 A6 | A335 L2 A8 A11 A13 A7 A5 A4 A3 L1 | L80 A320 A323 A325 A319 A318 A316 A314 L79 A335 | A335 L4 A16 A19 A21 A15 A14 A12 A10 L3 | L78 A312 A315 A317 A311 A310 A308 A306 L77 A335 | A335 L6 A24 A27 A29 A23 A22 A20 A18 L5 | L76 A304 A307 A309 A303 A302 A300 A298 L75 A335 | A335 L8 A32 A35 A37 A31 A30 A28 A26 L7 | L74 A296 A299 A301 A295 A294 A292 A290 L73 A335 | A335 L10 A40 A43 A45 A39 A38 A36 A34 L9 | L72 A288 A291 A293 A287 A286 A284 A282 L71 A335 | A335 L12 A48 A51 A53 A47 A46 A44 A42 L11 | L70 A280 A283 A285 A279 A278 A276 A274 L69 A335 | A335 L14 A56 A59 A61 A55 A54 A52 A50 L13 | L68 A272 A275 A277 A271 A270 A268 A266 L67 A335 | A335 L16 A64 A67 A69 A63 A62 A60 A58 L15 | L66 A264 A267 A269 A263 A262 A260 A258 L65 A335 | A335 L18 A72 A75 A77 A71 A70 A68 A66 L17 | L64 A256 A259 A261 A255 A254 A252 A250 L63 A335 | A335 L20 A80 A83 A85 A79 A78 A76 A74 L19 | L62 A248 A251 A253 A247 A246 A244 A242 L61 A335 | A335 L22 A88 A91 A93 A87 A86 A84 A82 L21 | A335 L24 A96 A99 A101 A95 A94 A92 A90 L23 | L60 A240 A243 A245 A239 A238 A236 A234 L59 A335 | A335 L26 A104 A107 A109 A103 A102 A100 A98 L25 | L58 A232 A235 A237 A231 A230 A228 A226 L57 A335 | A335 L28 A112 A115 A117 A111 A110 A108 A106 L27 | L56 A224 A227 A229 A223 A222 A220 A218 L55 A335 | A335 L30 A120 A123 A125 A119 A118 A116 A114 L29 | L54 A216 A219 A221 A215 A214 A212 A210 L53 A335 | A335 L32 A128 A131 A133 A127 A126 A124 A122 L31 | L52 A208 A211 A213 A207 A206 A204 A202 L51 A335 | A335 L34 A136 A139 A141 A135 A134 A132 A130 L33 | L50 A200 A203 A205 A199 A198 A196 A194 L49 A335 | A335 L36 A144 A147 A149 A143 A142 A140 A138 L35 | L48 A192 A195 A197 A191 A190 A188 A186 L47 A335 | A335 L38 A152 A155 A157 A151 A150 A148 A146 L37 | L46 A184 A187 A189 A183 A182 A180 A178 L45 A335 | A335 L40 A160 A163 A165 A159 A158 A156 A154 L39 | L44 A176 A179 A181 A175 A174 A172 A170 L43 A335 | A335 L42 A168 A171 A173 A167 A166 A164 A162 L41 | L83 A347 L94 A339 A328 | A328 A339 L95 A347 L83 | A328 A336 A350 A339 | A339 A351 A337 A328 | A347 L95 A339 L94 | A328 L82 A333 L85 A336 | A337 L92 A334 L91 A328 | A328 A336 L86 A333 L82 | L95 A340 L94 A339 | A337 A352 A338 A328 | A328 A338 A349 A336 | A333 L86 A329 L82 | L82 A329 L85 A333 | L95 A348 L94 A340 | A338 L89 A343 L88 A328 | L86 A336 L85 A333 | A333 L85 A329 L86 | A336 L86 A340 L85 | A340 L86 A342 L85 | L91 A334 L92 A337 | A337 L92 A340 L91 | L92 A346 L91 A340 | L89 A340 L88 A338 | A338 L88 A343 L89 | L91 A331 L92 A334 | A334 L92 A331 L91 | A340 L89 A344 L88
fillet "フィレット1" radius 1.05 16 edges at (1.2276, 17.8793, 2) (1.2276, 11.957, 2) (-6.4292, 2.8974, 2) (-13.7543, 2.8974, 2) (-13.7543, -0.1026, 2) (-6.4292, -0.1026, 2) (1.2276, -9.1622, 2) (1.2276, -15.0844, 2) (4.2276, -15.0844, 2) (4.2276, -9.1622, 2) (11.8843, -0.1026, 2) (19.2094, -0.1026, 2) (19.2094, 2.8974, 2) (11.8843, 2.8974, 2) (4.2276, 11.957, 2) (4.2276, 17.8793, 2)
sketch "スケッチ2" plane through (0, 0, 0) normal (0, 0, -1) x (-1, 0, 0)
  circle A0 centre (-2.7276, -4.6026) radius 1.5 projected
  point P0 (0, 0)
  constraints: 1 coincident
hole "穴1" at (2.7276, -4.6026, 0) direction (0, 0, 1) diameter 3 end through all countersink diameter 6 countersink angle 90
chamfer "面取り4" distance 1.5 angle 45 1 edges at (1.2276, 7.3974, 0)
